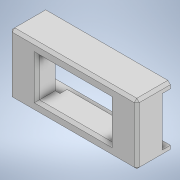
# Autodesk Inventor part: Part1
Saved by Autodesk Inventor 2021 (Build 250183000, 183)
## iProperties
Created: 2020-08-04
Part Number: Part1
Material: Generic
Document SubType Name: Modeling
Designer: CASE-SMALL2
Density: 1 g/cm^3
Appearance: Default
Author: CASE-SMALL2
Autodesk Inventor part; units mm, degrees
ref_plane "YZ Plane" through (0, 0, 0) normal (1, 0, 0) x (0, 1, 0)
ref_plane "XZ Plane" through (0, 0, 0) normal (0, 1, 0) x (-1, 0, 0)
ref_plane "XY Plane" through (0, 0, 0) normal (0, 0, 1) x (1, 0, 0)
sketch "Sketch1" plane through (0, 0, 0) normal (0, 0, 1) x (1, 0, 0)
  line L0 (-7.15, -3.85) -> (7.15, -3.85)
  line L1 (7.15, -3.85) -> (7.15, 3.85)
  line L2 (7.15, 3.85) -> (-7.15, 3.85)
  line L3 (-7.15, 3.85) -> (-7.15, -3.85)
  line L4 (-7.15, -3.85) -> (7.15, 3.85) construction
  line L5 (7.15, -3.85) -> (-7.15, 3.85) construction
  line L6 (-12.5, -6) -> (12.5, -6)
  line L7 (12.5, -6) -> (12.5, 6)
  line L8 (12.5, 6) -> (-12.5, 6)
  line L9 (-12.5, 6) -> (-12.5, -6)
  line L10 (-12.5, -6) -> (12.5, 6) construction
  line L11 (12.5, -6) -> (-12.5, 6) construction
  point P0 (0, 0)
  dimension "d0" = 7.7
  dimension "d1" = 14.3
  dimension "d3" = 12
  dimension "d4" = 25
  constraints: 24 end point, 4 midpoint, 4 parallel, 2 horizontal, 2 perpendicular
  measures "d0" distance between parallel lines of L0 L2
  measures "d1" distance between parallel lines of L1 L3
  measures "d3" distance between parallel lines of L6 L8
  measures "d4" distance between parallel lines of L7 L9
extrude "Extrusion1" add sketch "Sketch1" along normal blind 6.6
sketch "Sketch2" plane through (0, 0, 0) normal (0, 0, -1) x (-1, 0, 0)
  line L0 (10.15, 4.8) -> (7.15, 4.8)
  line L1 (7.15, 4.8) -> (7.15, -4.8)
  line L2 (7.15, -4.8) -> (10.15, -4.8)
  line L3 (10.15, -4.8) -> (10.15, 4.8)
  line L4 (7.15, 3.85) -> (-7.15, 3.85) projected
  line L5 (-7.15, -3.85) -> (7.15, -3.85) projected
  point P0 (0, 0)
  dimension "d8" = 3
  dimension "d18" = 9.6
  dimension "d19" = 0.95
  constraints: 8 end point, 2 parallel, 1 horizontal, 1 perpendicular, 1 point on line
  measures "d8" distance between parallel lines of L1 L3
  measures "d18" distance of L2.end L0.start
  measures "d19" distance between parallel lines of L4 L0
extrude "Extrusion2" cut sketch "Sketch2" against normal blind 3
sketch "Sketch3" plane through (0, 0, 0) normal (0, 0, -1) x (-1, 0, 0)
  line L0 (17.5, 0) -> (-17.5, 0) projected
  line L1 (-12.65, -4.8) -> (10.95, -4.8)
  line L2 (10.95, -4.8) -> (10.95, 4.8)
  line L3 (10.95, 4.8) -> (-12.65, 4.8)
  line L4 (-12.65, 4.8) -> (-12.65, -4.8)
  line L5 (-12.65, -4.8) -> (10.95, 4.8) construction
  line L6 (10.95, -4.8) -> (-12.65, 4.8) construction
  line L7 (-7.15, 3.85) -> (-7.15, -3.85) projected
  line L8 (7.15, -3.85) -> (7.15, 3.85) projected
  line L9 (10.15, 4.8) -> (10.15, -4.8) projected
  point P0 (0, 0)
  point P1 (-0.85, 0)
  dimension "d13" = 5.5
  dimension "d14" = 3.8
  dimension "d15" = 9.6
  constraints: 12 end point, 2 midpoint, 2 parallel, 1 horizontal, 1 perpendicular, 1 point on line
  measures "d13" distance between parallel lines of L7 L4
  measures "d14" distance between parallel lines of L8 L2
  measures "d15" distance between parallel lines of L1 L3
extrude "Extrusion3" cut sketch "Sketch3" against normal blind 1.6
chamfer "Chamfer1" distance 0.95 angle 45 4 edges at (-7.15, 3.85, 2.3) (-7.15, -3.85, 2.3) (-10.15, -4.8, 2.3) (-10.15, 4.8, 2.3)
chamfer "Chamfer2" distance 0.5 angle 45 12 edges at (0, 3.85, 6.6) (-7.15, 0, 6.6) (0, 6, 6.6) (-12.5, 0, 6.6) (0, -6, 6.6) (12.5, 0, 6.6) (7.15, 0, 6.6) (0, -3.85, 6.6) (-12.5, 6, 3.3) (12.5, 6, 3.3) (12.5, -6, 3.3) (-12.5, -6, 3.3)
body "Solid1"
